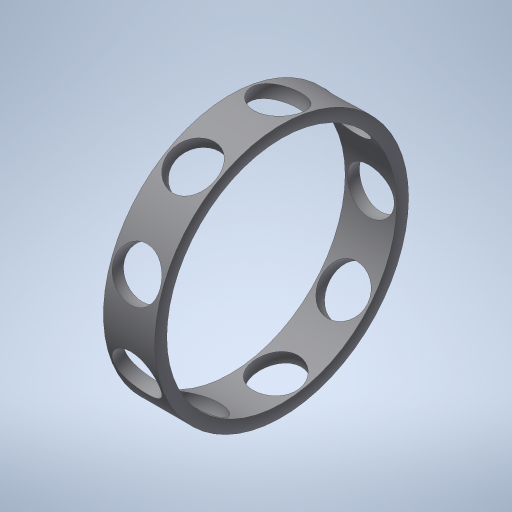
# Autodesk Inventor part: RF-2210X2HH_cage
Saved by Autodesk Inventor 2024.3 (Build 283343010, 343A)
## iProperties
Created: 2019-07-25
Part Number: RF-2210X2HH_cage
Material: 一般
Catalog Web Link: www.cadenas.de
Description: Radial Flanged Ball Bearings (RF-Series/LF series) Metric ST cage-Radial Flanged Ball Bearings (RF-Series/LF series) Metric Shielded Type
Vendor: NMB
Document SubType Name: Modeling
Designer: psadmin
Manufacturer: NMB
Mass: 0.08156 g
Surface Area: 3.56391 cm^2
Volume: 0.08156 cm^3
Density: 1 g/cm^3
Appearance: PSOLRGB-192-192-192
Category: PARTsolutions
Company: NMB
PSOL_IDENT_0: {$CADENAS_DATA\23d-libs\nmb\pbbp\radial_flanged_ball_bearings\rfbb_rflfs_m\rflf_shielded_cage.prj},2
PSOL_IDENT_1: 33 {VTYP=3D},{NB=RF-2210X2HH_cage},{LINA=RF-2210X2HH_cage},{NN=Radial Flanged Ball Bearings (RF-Seri
PSOL_IDENT_2: es/LF series) Metric ST cage},{DATE=11.11.2013 05:13:45},{GEOMDATE=24.10.2013 10:21:00},{VERSION=},{
PSOL_IDENT_3: LINEID=1560},{WBVAR=},{WBNUMERIC=}  {NB=RF-2210X2HH_cage},{LINA=RF-2210X2HH_cage},{KT=DUMMY},{IDNR=}
PSOL_IDENT_4: ,{PN=RF-2210X2HH},{SHLD=shielded},{FLANG=flanged},{SD=10.000},{D=22.000},{B=6.000},{SR=0.30},{BCZ=9}
PSOL_IDENT_5: ,{DW=3.1750},{LI=12.40},{LO=19.08},{D1=25.000},{C1=1.50},{D2=0.0},{C2=0.00},{COR=1273},{CR=1065},{PC
PSOL_IDENT_6: D=16.000},{U=19.175},{W=12.825},{Y=1.588},{Z=1.588},{AA=18.858},{AC=1.20},{AD=0.000},{AF=0.00},{AQ=0
PSOL_IDENT_7: .20},{AH=19.28},{AI=12.60},{AJ=0.40}
NN: Radial Flanged Ball Bearings (RF-Series/LF series) Metric ST cage
NT: Radial Flanged Ball Bearings (RF-Series/LF series) Metric Shielded Type
NB: RF-2210X2HH_cage
NBSYN: $PN._cage
LINA: RF-2210X2HH_cage
PN: RF-2210X2HH
SHLD: shielded
FLANG: flanged
SD: 10
D: 22
B: 6
SR: 0.3
BCZ: 9
DW: 3.175
LI: 12.4
LO: 19.08
D1: 25
C1: 1.5
D2: 0
C2: 0
COR: 1273
CR: 1065
PCD: 16
U: 19.175
W: 12.825
Y: 1.588
Z: 1.588
AA: 18.858
AC: 1.2
AD: 0
AF: 0
AQ: 0.2
AH: 19.28
AI: 12.6
AJ: 0.4
SUPPLIER: NMB
ARTICLENO: RF-2210X2HH_cage
BOMINFO: RF-2210X2HH_cage
CREATOR: CADENAS GmbH
Title: RF-2210X2HH_cage
Author: Cadenas PARTsolutions
Comments: Radial Flanged Ball Bearings (RF-Series/LF series) Metric Shielded Type
Autodesk Inventor part; units mm, degrees
note: some values were not read from the file. Chosen so that the rebuilt part matches the saved one: pattern direction of "Circular Pattern1".
sketch "Sketch_6" plane through (0, 0, 0) normal (0, 0, 1) x (1, 0, 0)
  line L0 (4.7006, 0) -> (1.2994, 0)
  arc A0 (1.2994, 8.3969) -> (1.2994, 7.6031) centre (3, 8) ccw
  line L1 (1.2994, 7.6031) -> (4.7006, 7.6031)
  arc A1 (4.7006, 7.6031) -> (4.7006, 8.3969) centre (3, 8) ccw
  line L2 (4.7006, 8.3969) -> (1.2994, 8.3969)
  constraints: 6 end point, 4 point on circle, 2 centre point
revolve "Revolution1" add sketch "Sketch_6" angle 360 about axis through (4.7006, 0, 0) along (1, 0, 0)
sketch "Sketch_2" plane through (3, 0, 0) normal (1, 0, 0) x (0, 0, -1)
  line L0 (1.6034, 8) -> (-1.6034, 8)
  arc A0 (1.6034, 8) -> (-1.6034, 8) centre (0, 8) ccw
  line L1 (1.6034, 8) -> (-1.6034, 8)
  constraints: 4 end point, 2 point on circle, 1 centre point
revolve "Revolution2" cut sketch "Sketch_2" angle 360 about axis through (3, 8, -1.6034) along (0, 0, -1)
pattern_circular "Circular Pattern1" count 9 over 360 about axis through (3, 0, 0) along (1, 0, 0) of "Revolution2"
ref_plane "1_XY" through (3, 0, 0) normal (1, 0, 0) x (0, 0, -1)
ref_plane "1_YZ" through (3, 0, 0) normal (0, 0, -1) x (0, 1, 0)
ref_plane "1_ZX" through (3, 0, 0) normal (0, 1, 0) x (1, 0, 0)
ref_plane "2_1_XY" through (3, 8, 0) normal (1, 0, 0) x (0, 0, -1)
ref_plane "2_1_YZ" through (3, 8, 0) normal (0, 0, -1) x (0, 1, 0)
ref_plane "2_1_ZX" through (3, 8, 0) normal (0, 1, 0) x (1, 0, 0)
ref_plane "2_2_XY" through (3, 6.1284, 5.1423) normal (1, 0, 0) x (0, 0, -1)
ref_plane "2_2_YZ" through (3, 6.1284, 5.1423) normal (0, 0, -1) x (0, 1, 0)
ref_plane "2_2_ZX" through (3, 6.1284, 5.1423) normal (0, 1, 0) x (1, 0, 0)
ref_plane "2_3_XY" through (3, 1.3892, 7.8785) normal (1, 0, 0) x (0, 0, -1)
ref_plane "2_3_YZ" through (3, 1.3892, 7.8785) normal (0, 0, -1) x (0, 1, 0)
ref_plane "2_3_ZX" through (3, 1.3892, 7.8785) normal (0, 1, 0) x (1, 0, 0)
ref_plane "2_4_XY" through (3, -4, 6.9282) normal (1, 0, 0) x (0, 0, -1)
ref_plane "2_4_YZ" through (3, -4, 6.9282) normal (0, 0, -1) x (0, 1, 0)
ref_plane "2_4_ZX" through (3, -4, 6.9282) normal (0, 1, 0) x (1, 0, 0)
ref_plane "2_5_XY" through (3, -7.5175, 2.7362) normal (1, 0, 0) x (0, 0, -1)
ref_plane "2_5_YZ" through (3, -7.5175, 2.7362) normal (0, 0, -1) x (0, 1, 0)
ref_plane "2_5_ZX" through (3, -7.5175, 2.7362) normal (0, 1, 0) x (1, 0, 0)
ref_plane "2_6_XY" through (3, -7.5175, -2.7362) normal (1, 0, 0) x (0, 0, -1)
ref_plane "2_6_YZ" through (3, -7.5175, -2.7362) normal (0, 0, -1) x (0, 1, 0)
ref_plane "2_6_ZX" through (3, -7.5175, -2.7362) normal (0, 1, 0) x (1, 0, 0)
ref_plane "2_7_XY" through (3, -4, -6.9282) normal (1, 0, 0) x (0, 0, -1)
ref_plane "2_7_YZ" through (3, -4, -6.9282) normal (0, 0, -1) x (0, 1, 0)
ref_plane "2_7_ZX" through (3, -4, -6.9282) normal (0, 1, 0) x (1, 0, 0)
ref_plane "2_8_XY" through (3, 1.3892, -7.8785) normal (1, 0, 0) x (0, 0, -1)
ref_plane "2_8_YZ" through (3, 1.3892, -7.8785) normal (0, 0, -1) x (0, 1, 0)
ref_plane "2_8_ZX" through (3, 1.3892, -7.8785) normal (0, 1, 0) x (1, 0, 0)
ref_plane "2_9_XY" through (3, 6.1284, -5.1423) normal (1, 0, 0) x (0, 0, -1)
ref_plane "2_9_YZ" through (3, 6.1284, -5.1423) normal (0, 0, -1) x (0, 1, 0)
ref_plane "2_9_ZX" through (3, 6.1284, -5.1423) normal (0, 1, 0) x (1, 0, 0)
body "Solid1"
